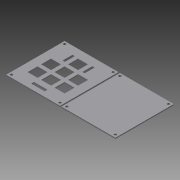
# Autodesk Inventor part: prototype_simple
Saved by Autodesk Inventor 2015 (Build 190159000, 159)
## iProperties
Created: 2015-07-10
Part Number: prototype_simple
Material: Generic
Document SubType Name: Modeling
Designer: Ben
Density: 1 g/cm^3
Appearance: Default
Author: Ben
Autodesk Inventor part; units mm, degrees
ref_plane "YZ Plane" through (0, 0, 0) normal (1, 0, 0) x (0, 1, 0)
ref_plane "XZ Plane" through (0, 0, 0) normal (0, 1, 0) x (-1, 0, 0)
ref_plane "XY Plane" through (0, 0, 0) normal (0, 0, 1) x (1, 0, 0)
sketch "1u" plane through (0, 0, 0) normal (0, 1, 0) x (-1, 0, 0)
  line L0 (7, 7) -> (-7, 7)
  line L1 (-7, 7) -> (-7, 6.4)
  line L2 (-7, 6.4) -> (-7.8, 6.4)
  line L3 (-7.8, 6.4) -> (-7.8, -6.4)
  line L4 (-7.8, -6.4) -> (-7, -6.4)
  line L5 (-7, -6.4) -> (-7, -7)
  line L6 (-7, -7) -> (7, -7)
  line L7 (7, -7) -> (7, -6.4)
  line L8 (7, -6.4) -> (7.8, -6.4)
  line L9 (7.8, -6.4) -> (7.8, 6.4)
  line L10 (7.8, 6.4) -> (7, 6.4)
  line L11 (7, 6.4) -> (7, 7)
  line L12 (9.525, -9.525) -> (9.525, 9.525) construction
  line L13 (9.525, 9.525) -> (-9.525, 9.525) construction
  line L14 (-9.525, 9.525) -> (-9.525, -9.525) construction
  line L15 (-9.525, -9.525) -> (9.525, -9.525) construction
  line L16 (9.525, 0) -> (7.8, 0) construction
  line L17 (-7.8, 0) -> (-9.525, 0) construction
  line L18 (0, 7) -> (0, 9.525) construction
  line L19 (0, -7) -> (0, -9.525) construction
  dimension "d0" = 12.8
  dimension "d1" = 14
  dimension "d2" = 14
  dimension "d3" = 15.6
  dimension "d4" = 19.05
  dimension "d5" = 19.05
  constraints: 40 end point, 14 perpendicular, 8 midpoint, 7 point on line, 6 collinear, 1 horizontal, 1 parallel, 1 vertical
  measures "d0" distance of L8.end L9.end
  measures "d1" distance between parallel lines of L0 L6
  measures "d2" distance of L5.end L6.end
  measures "d3" distance between parallel lines of L3 L9
  measures "d4" distance of L14.end L12.start
  measures "d5" distance of L12.start L12.end
sketch "1.25u" plane through (0, 0, 0) normal (0, 1, 0) x (-1, 0, 0)
  line L0 (7, 7) -> (-7, 7)
  line L1 (-7, 7) -> (-7, 6.4)
  line L2 (-7, 6.4) -> (-7.8, 6.4)
  line L3 (-7.8, 6.4) -> (-7.8, -6.4)
  line L4 (-7.8, -6.4) -> (-7, -6.4)
  line L5 (-7, -6.4) -> (-7, -7)
  line L6 (-7, -7) -> (7, -7)
  line L7 (7, -7) -> (7, -6.4)
  line L8 (7, -6.4) -> (7.8, -6.4)
  line L9 (7.8, -6.4) -> (7.8, 6.4)
  line L10 (7.8, 6.4) -> (7, 6.4)
  line L11 (7, 6.4) -> (7, 7)
  line L12 (11.9063, -9.525) -> (11.9063, 9.525) construction
  line L13 (11.9063, 9.525) -> (-11.9062, 9.525) construction
  line L14 (-11.9062, 9.525) -> (-11.9062, -9.525) construction
  line L15 (-11.9062, -9.525) -> (11.9063, -9.525) construction
  line L16 (11.9062, 0) -> (7.8, 0) construction
  line L17 (-7.8, 0) -> (-11.9062, 0) construction
  line L18 (0, 7) -> (0, 9.525) construction
  line L19 (0, -7) -> (0, -9.525) construction
  dimension "d45" = 12.8
  dimension "d46" = 14
  dimension "d47" = 14
  dimension "d48" = 15.6
  dimension "d49" = 23.8125
  dimension "d50" = 19.05
  constraints: 40 end point, 14 perpendicular, 8 midpoint, 7 point on line, 6 collinear, 1 horizontal, 1 parallel, 1 vertical
  measures "d45" distance of L8.end L9.end
  measures "d46" distance between parallel lines of L0 L6
  measures "d47" distance of L5.end L6.end
  measures "d48" distance between parallel lines of L3 L9
  measures "d49" distance of L14.end L12.start
  measures "d50" distance of L12.start L12.end
sketch "1.5u" plane through (0, 0, 0) normal (0, 1, 0) x (-1, 0, 0)
  line L0 (7, 7) -> (-7, 7)
  line L1 (-7, 7) -> (-7, 6.4)
  line L2 (-7, 6.4) -> (-7.8, 6.4)
  line L3 (-7.8, 6.4) -> (-7.8, -6.4)
  line L4 (-7.8, -6.4) -> (-7, -6.4)
  line L5 (-7, -6.4) -> (-7, -7)
  line L6 (-7, -7) -> (7, -7)
  line L7 (7, -7) -> (7, -6.4)
  line L8 (7, -6.4) -> (7.8, -6.4)
  line L9 (7.8, -6.4) -> (7.8, 6.4)
  line L10 (7.8, 6.4) -> (7, 6.4)
  line L11 (7, 6.4) -> (7, 7)
  line L12 (14.2875, -9.525) -> (14.2875, 9.525) construction
  line L13 (14.2875, 9.525) -> (-14.2875, 9.525) construction
  line L14 (-14.2875, 9.525) -> (-14.2875, -9.525) construction
  line L15 (-14.2875, -9.525) -> (14.2875, -9.525) construction
  line L16 (14.2875, 0) -> (7.8, 0) construction
  line L17 (-7.8, 0) -> (-14.2875, 0) construction
  line L18 (0, 7) -> (0, 9.525) construction
  line L19 (0, -7) -> (0, -9.525) construction
  dimension "d39" = 12.8
  dimension "d40" = 14
  dimension "d41" = 14
  dimension "d42" = 15.6
  dimension "d43" = 28.575
  dimension "d44" = 19.05
  constraints: 40 end point, 14 perpendicular, 8 midpoint, 7 point on line, 6 collinear, 1 horizontal, 1 parallel, 1 vertical
  measures "d39" distance of L8.end L9.end
  measures "d40" distance between parallel lines of L0 L6
  measures "d41" distance of L5.end L6.end
  measures "d42" distance between parallel lines of L3 L9
  measures "d43" distance of L14.end L12.start
  measures "d44" distance of L12.start L12.end
sketch "2u" plane through (0, 0, 0) normal (0, 1, 0) x (-1, 0, 0)
  line L0 (7, -7) -> (7, -6.4)
  line L1 (7, -6.4) -> (7.8, -6.4)
  line L2 (19.05, 0) -> (7.8, 0) construction
  line L3 (19.05, -9.525) -> (19.05, 9.525) construction
  line L4 (7.8, -6.4) -> (7.8, 6.4)
  line L5 (0, -7) -> (0, -9.525) construction
  line L6 (-7, -6.4) -> (-7, -7)
  line L7 (-7.8, 0) -> (-19.05, 0) construction
  line L8 (-7.8, -6.4) -> (-7, -6.4)
  line L9 (0, 7) -> (0, 9.525) construction
  line L10 (7, 7) -> (-7, 7)
  line L11 (-7, -7) -> (7, -7)
  line L12 (-19.05, -9.525) -> (19.05, -9.525) construction
  line L13 (19.05, 9.525) -> (-19.05, 9.525) construction
  line L14 (-19.05, 9.525) -> (-19.05, -9.525) construction
  line L15 (-7, 7) -> (-7, 6.4)
  line L16 (-7, 6.4) -> (-7.8, 6.4)
  line L17 (-7.8, 6.4) -> (-7.8, -6.4)
  line L18 (7, 6.4) -> (7, 7)
  line L19 (7.8, 6.4) -> (7, 6.4)
  line L20 (15.6, -6.24) -> (15.6, 7.76)
  line L21 (15.6, 7.76) -> (12.4, 7.76)
  line L22 (12.4, 7.76) -> (12.4, -6.24)
  line L23 (12.4, -6.24) -> (15.6, -6.24)
  line L24 (14, -6.24) -> (14, 7.76) construction
  line L25 (15.6, 0.76) -> (12.4, 0.76) construction
  line L26 (-12.4, 7.76) -> (-12.4, -6.24)
  line L27 (-12.4, -6.24) -> (-15.6, -6.24)
  line L28 (-15.6, -6.24) -> (-15.6, 7.76)
  line L29 (-15.6, 7.76) -> (-12.4, 7.76)
  line L30 (-14, -6.24) -> (-14, 7.76) construction
  line L31 (-15.6, 0.76) -> (-12.4, 0.76) construction
  dimension "d28" = 12.8
  dimension "d29" = 14
  dimension "d30" = 14
  dimension "d31" = 15.6
  dimension "d32" = 38.1
  dimension "d33" = 19.05
  dimension "d34" = 3.2
  dimension "d35" = 14
  dimension "d36" = 14
  dimension "d37" = 0.76
  constraints: 64 end point, 17 perpendicular, 12 midpoint, 8 symmetric about line, 7 point on line, 6 collinear, 2 vertical, 1 horizontal, 1 parallel
  measures "d28" distance of L4.start L4.end
  measures "d29" distance between parallel lines of L10 L11
  measures "d30" distance of L11.start L0.start
  measures "d31" distance between parallel lines of L17 L4
  measures "d32" distance of L12.start L3.start
  measures "d33" distance of L3.start L3.end
  measures "d34" distance of L22.end L20.start
  measures "d35" distance of L20.start L21.start
  measures "d36" distance between parallel lines of L5 L24
  measures "d37" distance between parallel lines of L25 L2
sketch "Sketch11" plane through (0, 0, 0) normal (0, 1, 0) x (1, 0, 0)
  line L0 (86.4523, 62.3313) -> (72.4523, 62.3313)
  line L1 (72.4523, 48.3313) -> (86.4523, 48.3313)
  line L2 (88.9773, 45.8063) -> (88.9773, 64.8563) construction
  line L3 (88.9773, 64.8563) -> (69.9273, 64.8563) construction
  line L4 (69.9273, 64.8563) -> (69.9273, 45.8063) construction
  line L5 (69.9273, 45.8063) -> (88.9773, 45.8063) construction
  line L6 (117.5523, 64.8563) -> (117.5523, 83.9063) construction
  line L7 (79.4523, 64.8563) -> (117.5523, 64.8563) construction
  line L8 (117.5523, 83.9063) -> (79.4523, 83.9063) construction
  line L9 (98.5023, 81.3813) -> (98.5023, 83.9063) construction
  line L10 (98.5023, 67.3813) -> (98.5023, 64.8563) construction
  line L11 (91.5023, 67.3813) -> (105.5023, 67.3813)
  line L12 (105.5023, 81.3813) -> (91.5023, 81.3813)
  line L13 (82.9023, 82.1413) -> (86.1023, 82.1413)
  line L14 (114.1023, 82.1413) -> (110.9023, 82.1413)
  line L15 (110.9023, 82.1413) -> (110.9023, 68.1413)
  line L16 (112.5023, 68.1413) -> (112.5023, 82.1413) construction
  line L17 (114.1023, 68.1413) -> (114.1023, 82.1413)
  line L18 (114.1023, 75.1413) -> (110.9023, 75.1413) construction
  line L19 (110.9023, 68.1413) -> (114.1023, 68.1413)
  line L20 (82.9023, 75.1413) -> (86.1023, 75.1413) construction
  line L21 (86.1023, 82.1413) -> (86.1023, 68.1413)
  line L22 (84.5023, 68.1413) -> (84.5023, 82.1413) construction
  line L23 (82.9023, 68.1413) -> (82.9023, 82.1413)
  line L24 (79.4523, 83.9063) -> (79.4523, 64.8563) construction
  line L25 (86.1023, 68.1413) -> (82.9023, 68.1413)
  line L26 (67.9723, 85.8613) -> (129.0323, 85.8613) construction
  line L27 (129.0323, 85.8613) -> (129.0323, 18.4513) construction
  line L28 (129.0323, 18.4513) -> (67.9723, 18.4513) construction
  line L29 (67.9723, 18.4513) -> (67.9723, 85.8613) construction
  line L30 (98.5023, 85.8613) -> (98.5023, 83.9063) construction
  line L31 (60.4723, 93.3613) -> (136.5323, 93.3613)
  line L32 (136.5323, 93.3613) -> (136.5323, 10.9513)
  line L33 (136.5323, 10.9513) -> (60.4723, 10.9513)
  line L34 (60.4723, 10.9513) -> (60.4723, 93.3613)
  line L35 (98.5023, 93.3613) -> (98.5023, 85.8613) construction
  line L36 (136.5323, 52.1563) -> (129.0323, 52.1563) construction
  line L37 (60.4723, 52.1563) -> (67.9723, 52.1563) construction
  line L38 (98.5023, 10.9513) -> (98.5023, 18.4513) construction
  line L39 (88.9773, 21.7213) -> (108.0273, 21.7213)
  line L40 (108.0273, 21.7213) -> (108.0273, 17.7213)
  line L41 (108.0273, 17.7213) -> (88.9773, 17.7213)
  line L42 (88.9773, 17.7213) -> (88.9773, 21.7213)
  line L43 (88.9773, 19.7213) -> (108.0273, 19.7213) construction
  line L44 (64.2223, 89.6113) -> (132.7823, 89.6113) construction
  line L45 (132.7823, 89.6113) -> (132.7823, 14.7013) construction
  line L46 (132.7823, 14.7013) -> (64.2223, 14.7013) construction
  line L47 (64.2223, 14.7013) -> (64.2223, 89.6113) construction
  circle A0 centre (64.2223, 89.6113) radius 1.75
  circle A1 centre (132.7823, 89.6113) radius 1.75
  circle A2 centre (132.7823, 14.7013) radius 1.75
  circle A3 centre (64.2223, 14.7013) radius 1.75
  line L48 (67.9723, 93.3613) -> (67.9723, 89.6113) construction
  line L49 (67.9723, 85.8613) -> (67.9723, 89.6113) construction
  line L50 (67.9723, 85.8613) -> (64.2223, 85.8613) construction
  line L51 (64.2223, 85.8613) -> (60.4723, 85.8613) construction
  line L52 (129.0323, 85.8613) -> (132.7823, 85.8613) construction
  line L53 (132.7823, 85.8613) -> (136.5323, 85.8613) construction
  line L54 (129.0323, 18.4513) -> (129.0323, 14.7013) construction
  line L55 (129.0323, 14.7013) -> (129.0323, 10.9513) construction
  line L56 (72.4523, 62.3313) -> (72.4523, 48.3313)
  line L57 (86.4523, 48.3313) -> (86.4523, 62.3313)
  line L58 (91.5023, 81.3813) -> (91.5023, 67.3813)
  line L59 (105.5023, 67.3813) -> (105.5023, 81.3813)
  line L60 (105.5023, 62.3313) -> (91.5023, 62.3313)
  line L61 (91.5023, 48.3313) -> (105.5023, 48.3313)
  line L62 (108.0273, 45.8063) -> (108.0273, 64.8563) construction
  line L63 (108.0273, 64.8563) -> (88.9773, 64.8563) construction
  line L64 (88.9773, 64.8563) -> (88.9773, 45.8063) construction
  line L65 (88.9773, 45.8063) -> (108.0273, 45.8063) construction
  line L66 (91.5023, 62.3313) -> (91.5023, 48.3313)
  line L67 (105.5023, 48.3313) -> (105.5023, 62.3313)
  line L68 (124.5523, 62.3313) -> (110.5523, 62.3313)
  line L69 (110.5523, 48.3313) -> (124.5523, 48.3313)
  line L70 (127.0773, 45.8063) -> (127.0773, 64.8563) construction
  line L71 (127.0773, 64.8563) -> (108.0273, 64.8563) construction
  line L72 (108.0273, 64.8563) -> (108.0273, 45.8063) construction
  line L73 (108.0273, 45.8063) -> (127.0773, 45.8063) construction
  line L74 (110.5523, 62.3313) -> (110.5523, 48.3313)
  line L75 (124.5523, 48.3313) -> (124.5523, 62.3313)
  line L76 (86.4523, 43.2813) -> (72.4523, 43.2813)
  line L77 (72.4523, 29.2813) -> (86.4523, 29.2813)
  line L78 (88.9773, 26.7563) -> (88.9773, 45.8063) construction
  line L79 (88.9773, 45.8063) -> (69.9273, 45.8063) construction
  line L80 (69.9273, 45.8063) -> (69.9273, 26.7563) construction
  line L81 (69.9273, 26.7563) -> (88.9773, 26.7563) construction
  line L82 (72.4523, 43.2813) -> (72.4523, 29.2813)
  line L83 (86.4523, 29.2813) -> (86.4523, 43.2813)
  line L84 (105.5023, 43.2813) -> (91.5023, 43.2813)
  line L85 (91.5023, 29.2813) -> (105.5023, 29.2813)
  line L86 (108.0273, 26.7563) -> (108.0273, 45.8063) construction
  line L87 (108.0273, 45.8063) -> (88.9773, 45.8063) construction
  line L88 (88.9773, 45.8063) -> (88.9773, 26.7563) construction
  line L89 (88.9773, 26.7563) -> (108.0273, 26.7563) construction
  line L90 (91.5023, 43.2813) -> (91.5023, 29.2813)
  line L91 (105.5023, 29.2813) -> (105.5023, 43.2813)
  line L92 (124.5523, 43.2813) -> (110.5523, 43.2813)
  line L93 (110.5523, 29.2813) -> (124.5523, 29.2813)
  line L94 (127.0773, 26.7563) -> (127.0773, 45.8063) construction
  line L95 (127.0773, 45.8063) -> (108.0273, 45.8063) construction
  line L96 (108.0273, 45.8063) -> (108.0273, 26.7563) construction
  line L97 (108.0273, 26.7563) -> (127.0773, 26.7563) construction
  line L98 (110.5523, 43.2813) -> (110.5523, 29.2813)
  line L99 (124.5523, 29.2813) -> (124.5523, 43.2813)
  line L100 (138.5323, 10.9513) -> (214.5923, 10.9513)
  line L101 (214.5923, 10.9513) -> (214.5923, 93.3613)
  line L102 (214.5923, 93.3613) -> (138.5323, 93.3613)
  line L103 (138.5323, 93.3613) -> (138.5323, 10.9513)
  line L104 (142.2823, 14.7013) -> (210.8423, 14.7013) construction
  line L105 (210.8423, 14.7013) -> (210.8423, 89.6113) construction
  line L106 (210.8423, 89.6113) -> (142.2823, 89.6113) construction
  line L107 (142.2823, 89.6113) -> (142.2823, 14.7013) construction
  circle A4 centre (142.2823, 89.6113) radius 1.75
  circle A5 centre (142.2823, 14.7013) radius 1.75
  circle A6 centre (210.8423, 89.6113) radius 1.75
  circle A7 centre (210.8423, 14.7013) radius 1.75
  point P0 (0, 0)
  dimension "d299" = 14
  dimension "d300" = 14
  dimension "d302" = 19.05
  dimension "d303" = 19.05
  dimension "d313" = 14
  dimension "d314" = 14
  dimension "d316" = 38.1
  dimension "d317" = 19.05
  dimension "d318" = 3.2
  dimension "d319" = 14
  dimension "d320" = 14
  dimension "d323" = 61.06
  dimension "d324" = 67.41
  dimension "d325" = 7.5
  dimension "d326" = 1.27
  dimension "d327" = 4
  dimension "d328" = 3.5
  dimension "d329" = 3.5
  dimension "d330" = 3.5
  dimension "d331" = 3.5
  dimension "d358" = 1.955
  dimension "d359" = 2.525
  dimension "d361" = 2.525
  dimension "d362" = 1.765
  dimension "d363" = 1.955
  dimension "d364" = 21.005
  dimension "d365" = 19.05
  dimension "d366" = 60.4723
  dimension "d367" = 10.9513
  dimension "d370" = 19.05
  dimension "d373" = 19.05
  dimension "d382" = 2
  dimension "d383" = 3.75
  dimension "d384" = 3.75
  dimension "d385" = 3.75
  dimension "d386" = 3.75
  dimension "d387" = 3.5
  dimension "d388" = 3.5
  dimension "d389" = 3.5
  dimension "d390" = 3.5
  constraints: 216 end point, 26 perpendicular, 19 midpoint, 18 point on line, 15 parallel, 10 equal length, 9 horizontal, 8 centre point, 8 coincident, 8 symmetric about line, 5 vertical, 4 collinear, 78 other
  measures "d299" distance between parallel lines of L0 L1
  measures "d300" distance of L1.start L1.end
  measures "d302" distance of L4.end L2.start
  measures "d303" distance of L2.start L2.end
  measures "d313" distance between parallel lines of L12 L11
  measures "d314" distance of L11.start L11.end
  measures "d316" distance of L7.start L6.start
  measures "d317" distance of L6.start L6.end
  measures "d318" distance of L15.end L17.start
  measures "d319" distance of L17.start L14.start
  measures "d320" distance between parallel lines of L10 L16
  measures "d323" distance of L27.end L28.end
  measures "d324" distance of L26.end L27.end
  measures "d325" distance of L35.start L35.end
  measures "d326" distance between parallel lines of L28 L43
  measures "d327" distance between parallel lines of L41 L39
  measures "d328" diameter of A0
  measures "d329" diameter of A1
  measures "d330" diameter of A2
  measures "d331" diameter of A3
  measures "d358" distance of L30.start L9.end
  measures "d359" distance between parallel lines of L4 L56
  measures "d361" distance between parallel lines of L3 L0
  measures "d362" distance between parallel lines of L8 L14
  measures "d363" distance between parallel lines of L29 L4
  measures "d364" distance between parallel lines of L29 L42
  measures "d365" distance between parallel lines of L40 L42
  measures "d366" distance from line of point (0, 0) L34
  measures "d367" distance from line of point (0, 0) L33
  measures "d370" distance of L1.end L67.start
  measures "d373" distance of L1.end L83.start
  measures "d382" distance between parallel lines of L103 L32
  measures "d383" distance between parallel lines of L107 L103
  measures "d384" distance between parallel lines of L100 L104
  measures "d385" distance between parallel lines of L102 L106
  measures "d386" distance between parallel lines of L101 L105
  measures "d387" diameter of A4
  measures "d388" diameter of A5
  measures "d389" diameter of A6
  measures "d390" diameter of A7
extrude "Extrusion6" add sketch "Sketch11" along normal blind 1.5
body "Solid5"
